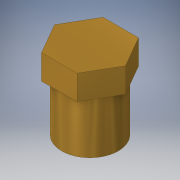
# Autodesk Inventor part: am-2024
Saved by Autodesk Inventor 2016 SP2 (Build 200236200, 236)
## iProperties
Created: 2017-03-30
Part Number: am-2024
Material: Brass
Document SubType Name: Modeling
Designer: smiku
Mass: 8.58114 g
Surface Area: 8.54184 cm^2
Volume: 1.01073 cm^3
Density: 8.49 g/cm^3
Appearance: Brass - Polished
Author: smiku
Autodesk Inventor part; units mm, degrees
ref_plane "YZ Plane" through (0, 0, 0) normal (1, 0, 0) x (0, 1, 0)
ref_plane "XZ Plane" through (0, 0, 0) normal (0, 1, 0) x (-1, 0, 0)
ref_plane "XY Plane" through (0, 0, 0) normal (0, 0, 1) x (1, 0, 0)
sketch "Sketch1" plane through (0, 0, 0) normal (0, 1, 0) x (-1, 0, 0)
  circle A0 centre (0, 0) radius 5.5372 construction
  line L0 (-3.1969, -5.5372) -> (-6.3938, 0)
  line L1 (-6.3938, 0) -> (-3.1969, 5.5372)
  line L2 (-3.1969, 5.5372) -> (3.1969, 5.5372)
  line L3 (3.1969, 5.5372) -> (6.3938, 0)
  line L4 (6.3938, 0) -> (3.1969, -5.5372)
  line L5 (3.1969, -5.5372) -> (-3.1969, -5.5372)
  point P0 (0, -5.5372)
  dimension "d0" = 11.0744
  constraints: 12 end point, 2 coincident, 1 horizontal, 1 midpoint, 1 vertical alignment, 15 other
extrude "Extrusion1" add sketch "Sketch1" along normal blind 4.445
sketch "Sketch2" plane through (0, 0, 0) normal (0, -1, 0) x (1, 0, 0)
  circle A0 centre (0, 0) radius 5.08
  circle A1 centre (0, 0) radius 2.794
  dimension "d3" = 10.16
  dimension "d4" = 5.588
  constraints: 2 centre point, 2 coincident
  measures "d3" diameter of A0
  measures "d4" diameter of A1
extrude "Extrusion2" add sketch "Sketch2" along normal blind 9.525
body "Solid1"
